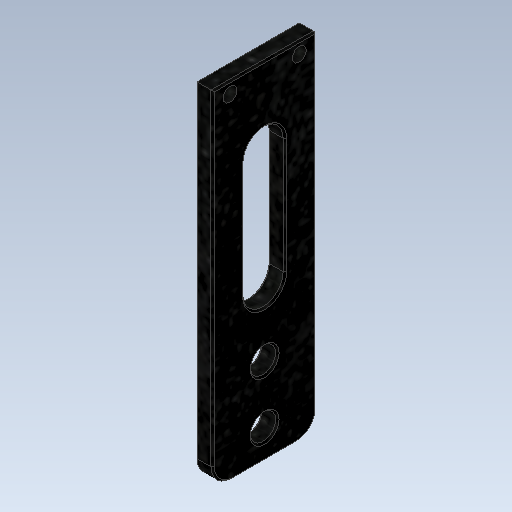
# Autodesk Inventor part: Ramka3
Saved by Autodesk Inventor 2020 (Build 240168000, 168)
## iProperties
Created: 2020-08-21
Part Number: Ramka3
Material: Steel
Document SubType Name: Modeling
Designer: estee
Density: 7.85 g/cm^3
Appearance: Plate
Author: estee
Autodesk Inventor part; units mm, degrees
ref_plane "YZ Plane" through (0, 0, 0) normal (1, 0, 0) x (0, 1, 0)
ref_plane "XZ Plane" through (0, 0, 0) normal (0, 1, 0) x (-1, 0, 0)
ref_plane "XY Plane" through (0, 0, 0) normal (0, 0, 1) x (1, 0, 0)
sketch "Sketch1" plane through (0, 0, 0) normal (1, 0, 0) x (0, 1, 0)
  line L0 (0, 0) -> (-60, 0)
  line L1 (-60, 0) -> (-60, -18)
  line L2 (-60, -18) -> (0, -18)
  line L3 (0, -18) -> (0, 0)
  line L4 (-13.5, -5.5) -> (-33.5, -5.5)
  line L5 (-37, -9) -> (-37, -9)
  line L6 (-33.5, -12.5) -> (-13.5, -12.5)
  line L7 (-10, -9) -> (-10, -9)
  arc A0 (-10, -9) -> (-13.5, -5.5) centre (-13.5, -9) ccw
  arc A1 (-13.5, -12.5) -> (-10, -9) centre (-13.5, -9) ccw
  arc A2 (-37, -9) -> (-33.5, -12.5) centre (-33.5, -9) ccw
  arc A3 (-33.5, -5.5) -> (-37, -9) centre (-33.5, -9) ccw
  point P0 (-37, -12.5)
  point P1 (-37, -5.5)
  point P2 (-10, -12.5)
  dimension "d0" = 60
  dimension "d1" = 18
  dimension "d2" = 27
  dimension "d3" = 7
  dimension "d4" = 5.5
  dimension "d5" = 10
  dimension "d6" = 3.5
  constraints: 16 end point, 8 point on circle, 8 tangent, 6 point on line, 4 centre point, 4 parallel, 3 equal radius, 2 horizontal, 2 perpendicular
  measures "d0" distance of L2.end L1.end
  measures "d1" distance of L2.end L0.start
  measures "d2" distance of point (-10, -12.5) point (-37, -12.5)
  measures "d3" distance of point (-37, -5.5) point (-37, -12.5)
  measures "d4" distance between parallel lines of L0 L4
  measures "d5" distance between parallel lines of L3 L7
  measures "d6" radius of A0
extrude "Extrusion1" add sketch "Sketch1" along normal blind 3
sketch "Sketch2" plane through (3, 0, 0) normal (1, 0, 0) x (0, 0, -1)
  line L0 (18, -60) -> (18, 0) projected
  line L1 (0, -60) -> (18, -60) projected
  point P0 (0, 0)
  point P1 (9, -45)
  point P2 (9, -55)
  dimension "d9" = 9
  dimension "d10" = 9
  dimension "d11" = 5
  dimension "d12" = 10
  measures "d9" distance from line of L0 point (9, -55)
  measures "d10" distance from line of L0 point (9, -45)
  measures "d11" distance from line of L1 point (9, -55)
  measures "d12" distance of point (9, -55) point (9, -45)
hole "Hole1" at (3, -45, -9) at (3, -55, -9) direction (-1, 0, 0) diameter 4.4 depth 8.8 tip angle 118
fillet "Fillet1" radius 3.5 2 edges at (1.5, -60, 0) (1.5, -60, -18)
chamfer "Chamfer1" distance 0.3 angle 45 25 edges at (3, 0, -9) (3, -28.25, -18) (3, -58.9749, -16.9749) (3, -60, -9) (3, -58.9749, -1.0251) (3, -28.25, 0) (1.5, 0, -18) (0, -28.25, -18) (0, -58.9749, -16.9749) (0, -60, -9) (0, -58.9749, -1.0251) (0, -28.25, 0) (0, 0, -9) (0, -10, -9) (0, -23.5, -5.5) (0, -37, -9) (0, -23.5, -12.5) (3, -23.5, -5.5) (3, -10, -9) (3, -23.5, -12.5) (3, -37, -9) (0, -55, -6.8) (0, -45, -6.8) (3, -55, -6.8) (3, -45, -6.8)
sketch "Sketch3" plane through (0, 0, 0) normal (-1, 0, 0) x (0, 0, 1)
  line L0 (-18, -0.3) -> (-18, -56.5) projected
  line L1 (0, -56.5) -> (0, 0) projected
  line L2 (0, 0) -> (-17.7, 0) projected
  point P0 (-15, -2)
  point P1 (-3, -2)
  dimension "d24" = 3
  dimension "d25" = 3
  dimension "d26" = 2
  dimension "d27" = 2
  measures "d24" distance from line of L0 point (-15, -2)
  measures "d25" distance from line of L1 point (-3, -2)
  measures "d26" distance from line of L2 point (-3, -2)
  measures "d27" distance from line of L2 point (-15, -2)
hole "Hole2" at (0, -2, -15) at (0, -2, -3) direction (1, 0, 0) diameter 2.4 depth 8.8 tip angle 118
body "Solid1"
